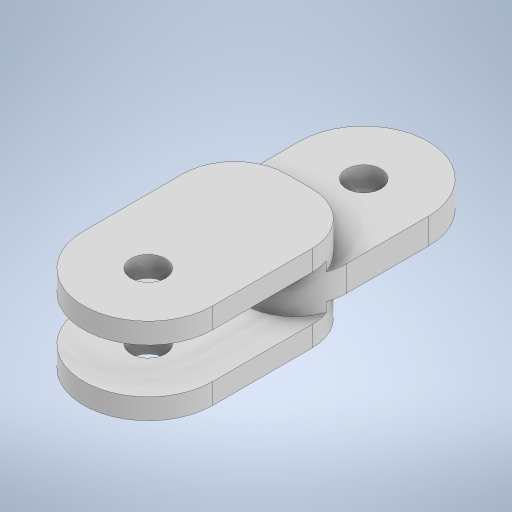
# Autodesk Inventor part: coupler
Saved by Autodesk Inventor 2024.2 (Build 282272000, 272)
## iProperties
Created: 2024-06-01
Part Number: coupler
Material: Generic
Document SubType Name: Modeling
Designer: Robin
Density: 1 g/cm^3
Appearance: Default
Author: Robin
Autodesk Inventor part; units mm, degrees
ref_plane "YZ Plane" through (0, 0, 0) normal (1, 0, 0) x (0, 1, 0)
ref_plane "XZ Plane" through (0, 0, 0) normal (0, 1, 0) x (-1, 0, 0)
ref_plane "XY Plane" through (0, 0, 0) normal (0, 0, 1) x (1, 0, 0)
sketch "Sketch1" plane through (0, 0, 0) normal (0, 1, 0) x (-1, 0, 0)
  line L0 (7.5, 20) -> (-7.5, 20)
  line L1 (-7.5, 20) -> (-7.5, -20)
  line L2 (-7.5, -20) -> (7.5, -20)
  line L3 (7.5, -20) -> (7.5, 20)
  circle A0 centre (0, -12.5) radius 7.5
  circle A1 centre (0, 12.5) radius 7.5
  circle A2 centre (0, 12.5) radius 2
  circle A3 centre (0, -12.5) radius 2
  point P0 (0, 0)
  point P1 (7.5, 0)
  point P2 (0, -20)
  point P3 (7.5, 12.5)
  point P4 (-7.5, 12.5)
  point P5 (-7.5, -12.5)
  point P6 (7.5, -12.5)
  dimension "d0" = 15
  dimension "d2" = 25
  dimension "d3" = 4
  dimension "d4" = 4
  constraints: 8 end point, 6 tangent, 4 centre point, 2 coincident, 2 midpoint, 2 parallel, 1 horizontal, 1 horizontal alignment, 1 perpendicular, 1 vertical alignment
  measures "d0" distance of L1.end L2.end
  measures "d2" distance of A0.centre A1.centre
  measures "d3" diameter of A3
  measures "d4" diameter of A2
extrude "Extrusion1" add sketch "Sketch1" along normal blind 10 contours A1 | L3 A0 L1 A1 | A0
sketch "Sketch2" plane through (7.5, 0, 12.5) normal (1, 0, 0) x (0, 0, -1)
  line L0 (-7.5, 0) -> (-7.5, 10) projected
  line L1 (-7.5, 7.6) -> (9.5, 7.6)
  line L2 (9.5, 7.6) -> (9.5, 2.4)
  line L3 (9.5, 2.4) -> (-7.5, 2.4)
  line L4 (-7.5, 2.4) -> (-7.5, 7.6)
  point P0 (12.5, 0)
  point P1 (-7.5, 5)
  point P2 (-7.5, 5)
  dimension "d7" = 17
  dimension "d8" = 5.2
  constraints: 8 end point, 2 midpoint, 2 parallel, 1 coincident, 1 horizontal, 1 perpendicular, 1 point on line
  measures "d7" distance of L2.end L3.end
  measures "d8" distance of L1.end L2.end
extrude "Extrusion2" cut sketch "Sketch2" against normal through all
fillet "Fillet1" radius 6 2 edges at (7.5, 5, 3) (-7.5, 5, 3)
sketch "Sketch4" plane through (7.5, 0, 12.5) normal (1, 0, 0) x (0, 0, -1)
  line L0 (32.5, 0) -> (32.5, 10) projected
  line L1 (32.5, 6.5) -> (17.5, 6.5)
  line L2 (17.5, 6.5) -> (17.5, 3.5)
  line L3 (17.5, 3.5) -> (32.5, 3.5)
  line L4 (32.5, 3.5) -> (32.5, 6.5)
  line L5 (15.5, 2.4) -> (15.5, 7.6) projected
  line L6 (0, 0) -> (25, 0) projected
  line L7 (32.5, 3.5) -> (17.5, 3.5)
  line L8 (17.5, 3.5) -> (17.5, 0)
  line L9 (17.5, 0) -> (32.5, 0)
  line L10 (32.5, 0) -> (32.5, 3.5)
  line L11 (25, 10) -> (0, 10) projected
  line L12 (32.5, 6.5) -> (17.5, 6.5)
  line L13 (17.5, 6.5) -> (17.5, 10)
  line L14 (17.5, 10) -> (32.5, 10)
  line L15 (32.5, 10) -> (32.5, 6.5)
  point P0 (12.5, 0)
  point P1 (17.5, 5)
  point P2 (15.5, 5)
  point P3 (17.5, 1.75)
  dimension "d15" = 3
  dimension "d16" = 15
  constraints: 24 end point, 6 parallel, 3 horizontal, 3 midpoint, 3 perpendicular, 3 point on line, 2 vertical alignment, 1 horizontal alignment
  measures "d15" distance between parallel lines of L1 L3
  measures "d16" distance of L2.end L3.end
extrude "Extrusion4" cut sketch "Sketch4" against normal through all contours L9 L6 L8 L3 L0 | L1 L13 L11 L14 L0
fillet "Fillet2" radius 6 4 edges at (7.5, 1.75, -5) (7.5, 8.25, -5) (-7.5, 1.75, -5) (-7.5, 8.25, -5)
body "Solid1"
